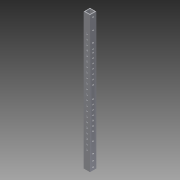
# Autodesk Inventor part: Chassis Part4 (26x28)
Saved by Autodesk Inventor 2013 (Build 170138000, 138)
## iProperties
Created: 2013-01-05
Part Number: Chassis Part4 (26x28)
Material: Aluminum 6061
Document SubType Name: Modeling
Designer: Moses
Density: 2.71 g/cm^3
Mass: 414.468 g
Surface Area: 998.032 cm^2
Volume: 152.94 cm^3
Author: Moses
Autodesk Inventor part; units mm, degrees
ref_plane "YZ Plane" through (0, 0, 0) normal (1, 0, 0) x (0, 1, 0)
ref_plane "XZ Plane" through (0, 0, 0) normal (0, 1, 0) x (-1, 0, 0)
ref_plane "XY Plane" through (0, 0, 0) normal (0, 0, 1) x (1, 0, 0)
sketch "Sketch1" plane through (0, 0, 0) normal (0, 1, 0) x (-1, 0, 0)
  line L0 (0, 25.4) -> (25.4, 25.4)
  line L1 (25.4, 25.4) -> (25.4, 0)
  line L2 (25.4, 0) -> (0, 0)
  line L3 (0, 0) -> (0, 25.4)
  line L4 (22.225, 22.225) -> (3.175, 22.225)
  line L5 (3.175, 22.225) -> (3.175, 3.175)
  line L6 (3.175, 3.175) -> (22.225, 3.175)
  line L7 (22.225, 3.175) -> (22.225, 22.225)
  dimension "d0" = 25.4
  dimension "d1" = 25.4
  dimension "d2" = 3.175
  constraints: 16 end point, 4 parallel, 2 perpendicular, 1 coincident, 1 horizontal, 3 other
  measures "d0" distance of L1.end L2.end
  measures "d1" distance of L0.end L1.end
  measures "d2" distance between parallel lines of L0 L4
extrude "Extrusion1" add sketch "Sketch1" along normal blind 558.8
sketch "Sketch2" plane through (-25.4, 0, 25.4) normal (0, 0, 1) x (1, 0, 0)
  line L0 (25.4, 0) -> (0, 0) projected
  line L1 (0, 558.8) -> (25.4, 558.8) projected
  line L2 (12.7, 558.8) -> (12.7, 0) construction
  line L3 (12.7, 0) -> (12.7, 13.97) construction
  circle A0 centre (12.7, 13.97) radius 3.302
  circle A1 centre (12.7, 33.6315) radius 3.302
  circle A2 centre (12.7, 53.293) radius 3.302
  circle A3 centre (12.7, 72.9544) radius 3.302
  circle A4 centre (12.7, 92.6159) radius 3.302
  circle A5 centre (12.7, 112.2774) radius 3.302
  circle A6 centre (12.7, 131.9389) radius 3.302
  circle A7 centre (12.7, 151.6004) radius 3.302
  circle A8 centre (12.7, 171.2619) radius 3.302
  circle A9 centre (12.7, 190.9233) radius 3.302
  circle A10 centre (12.7, 210.5848) radius 3.302
  circle A11 centre (12.7, 230.2463) radius 3.302
  circle A12 centre (12.7, 249.9078) radius 3.302
  circle A13 centre (12.7, 269.5693) radius 3.302
  circle A14 centre (12.7, 289.2307) radius 3.302
  circle A15 centre (12.7, 308.8922) radius 3.302
  circle A16 centre (12.7, 328.5537) radius 3.302
  circle A17 centre (12.7, 348.2152) radius 3.302
  circle A18 centre (12.7, 367.8767) radius 3.302
  circle A19 centre (12.7, 387.5381) radius 3.302
  circle A20 centre (12.7, 407.1996) radius 3.302
  circle A21 centre (12.7, 426.8611) radius 3.302
  circle A22 centre (12.7, 446.5226) radius 3.302
  circle A23 centre (12.7, 466.1841) radius 3.302
  circle A24 centre (12.7, 485.8456) radius 3.302
  circle A25 centre (12.7, 505.507) radius 3.302
  circle A26 centre (12.7, 525.1685) radius 3.302
  circle A27 centre (12.7, 544.83) radius 3.302
  dimension "d5" = 13.97
  dimension "d6" = 6.604
  dimension "d7" = 558.8
  dimension "d10" = 19.6615
  constraints: 28 centre point, 4 end point, 2 midpoint, 1 coincident, 1 point on line, 1 vertical, 54 other
  measures "d5" distance of L2.end L3.end
  measures "d6" diameter of A0
  measures "d7" distance of L0.end L1.start
  measures "d10" distance of A0.centre A1.centre
extrude "Extrusion2" cut sketch "Sketch2" against normal through all contours A3 | A4 | A5 | A6 | A7 | A8 | A9 | A10 | A11 | A12 | A13 | A14 | A15 | A16 | A17 | A18 | A19 | A20 | A21 | A22 | A23 | A24
sketch "Sketch3" plane through (-25.4, 0, 0) normal (-1, 0, 0) x (0, 0, 1)
  line L0 (25.4, 0) -> (25.4, 558.8) projected
  line L1 (0, 0) -> (0, 558.8) projected
  line L2 (0, 210.5848) -> (25.4, 210.5848) construction
  line L3 (12.7, 498.5456) -> (12.7, 454.0956) construction
  line L4 (12.7, 373.6152) -> (12.7, 322.8152) construction
  line L5 (12.7, 232.8098) -> (12.7, 188.3598) construction
  line L6 (12.7, 104.7044) -> (12.7, 60.2544) construction
  circle A0 centre (12.7, 498.5456) radius 3.302
  circle A1 centre (12.7, 454.0956) radius 3.302
  circle A2 centre (12.7, 373.6152) radius 3.302
  circle A3 centre (12.7, 322.8152) radius 3.302
  circle A4 centre (12.7, 232.8098) radius 3.302
  circle A5 centre (12.7, 188.3598) radius 3.302 construction
  circle A6 centre (12.7, 104.7044) radius 3.302
  circle A7 centre (12.7, 60.2544) radius 3.302
  line L7 (0, 279.4) -> (25.4, 279.4) construction
  line L8 (12.7, 304.8) -> (12.7, 254) construction
  circle A8 centre (12.7, 304.8) radius 3.302
  circle A9 centre (12.7, 254) radius 3.302
  line L9 (25.4, 0) -> (0, 0) projected
  line L10 (0, 558.8) -> (25.4, 558.8) projected
  circle A10 centre (12.7, 546.1) radius 3.302
  line L11 (12.7, 546.1) -> (12.7, 558.8) construction
  line L12 (12.7, 0) -> (12.7, 12.7) construction
  circle A11 centre (12.7, 12.7) radius 3.302
  line L13 (0, 82.4794) -> (25.4, 82.4794) construction
  line L14 (0, 476.3206) -> (25.4, 476.3206) construction
  line L15 (12.7, 12.7) -> (12.7, 34.8544) construction
  circle A12 centre (12.7, 34.8544) radius 3.302
  line L16 (0, 13.97) -> (25.4, 13.97) construction
  line L17 (0, 33.6315) -> (25.4, 33.6315) construction
  line L18 (0, 53.293) -> (25.4, 53.293) construction
  line L19 (0, 72.9544) -> (25.4, 72.9544) construction
  line L20 (0, 92.6159) -> (25.4, 92.6159) construction
  line L21 (0, 112.2774) -> (25.4, 112.2774) construction
  line L22 (0, 131.9389) -> (25.4, 131.9389) construction
  line L23 (0, 151.6004) -> (25.4, 151.6004) construction
  line L24 (0, 171.2619) -> (25.4, 171.2619) construction
  line L25 (0, 190.9233) -> (25.4, 190.9233) construction
  line L26 (0, 210.5848) -> (25.4, 210.5848) construction
  line L27 (0, 230.2463) -> (25.4, 230.2463) construction
  line L28 (0, 249.9078) -> (25.4, 249.9078) construction
  line L29 (0, 269.5693) -> (25.4, 269.5693) construction
  line L30 (0, 289.2307) -> (25.4, 289.2307) construction
  line L31 (0, 308.8922) -> (25.4, 308.8922) construction
  line L32 (0, 328.5537) -> (25.4, 328.5537) construction
  line L33 (0, 348.2152) -> (25.4, 348.2152) construction
  line L34 (0, 367.8767) -> (25.4, 367.8767) construction
  line L35 (0, 387.5381) -> (25.4, 387.5381) construction
  line L36 (0, 407.1996) -> (25.4, 407.1996) construction
  line L37 (0, 426.8611) -> (25.4, 426.8611) construction
  line L38 (0, 446.5226) -> (25.4, 446.5226) construction
  line L39 (0, 466.1841) -> (25.4, 466.1841) construction
  line L40 (0, 485.8456) -> (25.4, 485.8456) construction
  line L41 (0, 505.507) -> (25.4, 505.507) construction
  line L42 (0, 525.1685) -> (25.4, 525.1685) construction
  line L43 (0, 544.83) -> (25.4, 544.83) construction
  line L44 (3.175, 489.1476) -> (3.175, 482.5436) projected
  line L45 (3.175, 351.5172) -> (3.175, 344.9132) projected
  line L46 (3.175, 76.2564) -> (3.175, 69.6524) projected
  line L47 (3.175, 213.8868) -> (3.175, 207.2828) projected
  point P0 (12.7, 279.4)
  point P1 (12.7, 82.4794)
  point P2 (12.7, 476.3206)
  point P3 (12.7, 348.2152)
  point P4 (12.7, 210.5848)
  dimension "d17" = 44.45
  dimension "d18" = 50.8
  dimension "d19" = 44.45
  dimension "d20" = 44.45
  dimension "d21" = 6.604
  dimension "d22" = 6.604
  dimension "d23" = 6.604
  dimension "d24" = 6.604
  dimension "d25" = 6.604
  dimension "d26" = 6.604
  dimension "d27" = 6.604
  dimension "d28" = 6.604
  dimension "d31" = 50.8
  dimension "d32" = 6.604
  dimension "d33" = 6.604
  dimension "d40" = 12.7
  dimension "d41" = 6.604
  dimension "d42" = 12.7
  dimension "d43" = 6.604
  dimension "d64" = 25.4
  dimension "d65" = 6.604
  dimension "d66" = 13.97
  dimension "d67" = 558.8
  dimension "d70" = 19.6615
  dimension "d76" = 9.525
  dimension "d77" = 9.525
  constraints: 80 end point, 15 midpoint, 13 centre point, 12 coincident, 8 point on line, 5 collinear, 5 perpendicular, 3 vertical, 81 other
  measures "d17" distance of L3.start L3.end
  measures "d18" distance of L4.start L4.end
  measures "d19" distance of L5.start L5.end
  measures "d20" distance of L6.start L6.end
  measures "d21" diameter of A0
  measures "d22" diameter of A1
  measures "d23" diameter of A2
  measures "d24" diameter of A3
  measures "d25" diameter of A4
  measures "d26" diameter of A5
  measures "d27" diameter of A6
  measures "d28" diameter of A7
  measures "d31" distance of L8.start L8.end
  measures "d32" diameter of A8
  measures "d33" diameter of A9
  measures "d40" distance from line of L10 L11.start
  measures "d41" diameter of A10
  measures "d42" distance of L12.start L12.end
  measures "d43" diameter of A11
  measures "d64" distance of L6.end L15.end
  measures "d65" diameter of A12
  measures "d66" distance between parallel lines of L9 L16
  measures "d67" distance of L1.start L1.end
  measures "d70" distance of L16.start L17.start
  measures "d76" distance between parallel lines of L40 L14
  measures "d77" distance between parallel lines of L19 L13
extrude "Extrusion3" cut sketch "Sketch3" against normal through all contours A0 | A1 | A6 | A7 | A8 | A9 | A10 | A11 | A12
sketch "Sketch4" plane through (0, 0, 25.4) normal (1, 0, 0) x (0, 0, -1)
  circle A0 centre (12.7, 304.8) radius 3.302 construction
  circle A1 centre (12.7, 254) radius 3.302 construction
  line L0 (0, 0) -> (0, 558.8) projected
  line L1 (12.7, 304.8) -> (12.7, 323.85) construction
  line L2 (12.7, 254) -> (12.7, 234.95) construction
  circle A2 centre (12.7, 323.85) radius 3.302
  circle A3 centre (12.7, 234.95) radius 3.302
  line L3 (25.4, 0) -> (0, 0) projected
  line L4 (0, 558.8) -> (25.4, 558.8) projected
  line L5 (12.7, 558.8) -> (12.7, 0) construction
  circle A4 centre (12.7, 419.1) radius 3.302
  circle A5 centre (12.7, 400.05) radius 3.302
  circle A6 centre (12.7, 381) radius 3.302
  circle A7 centre (12.7, 361.95) radius 3.302
  circle A8 centre (12.7, 342.9) radius 3.302
  circle A9 centre (12.7, 431.8) radius 3.302
  circle A10 centre (12.7, 215.9) radius 3.302
  circle A11 centre (12.7, 196.85) radius 3.302
  circle A12 centre (12.7, 177.8) radius 3.302
  circle A13 centre (12.7, 158.75) radius 3.302
  circle A14 centre (12.7, 139.7) radius 3.302
  dimension "d46" = 19.05
  dimension "d47" = 19.05
  dimension "d48" = 6.604
  dimension "d49" = 6.604
  dimension "d52" = 6.604
  dimension "d53" = 139.7
  dimension "d80" = 19.05
  dimension "d85" = 12.7
  dimension "d88" = 19.05
  constraints: 13 centre point, 6 end point, 2 coincident, 2 midpoint, 2 point on line, 2 vertical, 1 collinear, 1 equal radius, 1 parallel, 18 other
  measures "d46" distance of L1.start L1.end
  measures "d47" distance of L2.start L2.end
  measures "d48" diameter of A2
  measures "d49" diameter of A3
  measures "d52" diameter of A4
  measures "d53" distance from line of L4 A4.centre
  measures "d80" distance of A4.centre A5.centre
  measures "d85" distance of A4.centre A9.centre
  measures "d88" distance of A3.centre A10.centre
extrude "Extrusion4" cut sketch "Sketch4" against normal blind 25.4
equation "\"d19\" = d17"
equation "\"d20\" = d17"
equation "\"d22\" = d21"
equation "\"d23\" = d21"
equation "\"d24\" = d21"
equation "\"d25\" = d21"
equation "\"d26\" = d21"
equation "\"d27\" = d21"
equation "\"d28\" = d21"
equation "\"d31\" = d18"
equation "\"d32\" = d21"
equation "\"d33\" = d21"
equation "\"d41\" = d21"
equation "\"d42\" = d40"
equation "\"d43\" = d21"
equation "\"d70\" = -0.0740741 * d66 + 0.037037 * d67"
equation "\"d76\" = d77"
body "Solid1"
